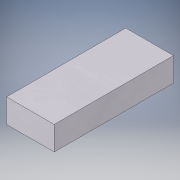
# Autodesk Inventor part: Shaker
Saved by Autodesk Inventor 2017 (Build 210142000, 142)
## iProperties
Created: 2016-12-09
Part Number: Shaker
Material: Aluminum 6061, Welded
Document SubType Name: Modeling
Designer: qupec
Density: 2.7 g/cm^3
Appearance: Weld - Aluminum
Author: qupec
Autodesk Inventor part; units mm, degrees
ref_plane "YZ Plane" through (0, 0, 0) normal (1, 0, 0) x (0, 1, 0)
ref_plane "XZ Plane" through (0, 0, 0) normal (0, 1, 0) x (-1, 0, 0)
ref_plane "XY Plane" through (0, 0, 0) normal (0, 0, 1) x (1, 0, 0)
sketch "Sketch1" plane through (0, 0, 0) normal (0, 1, 0) x (-1, 0, 0)
  line L0 (3, 7.5) -> (-3, 7.5)
  line L1 (-3, 7.5) -> (-3, -7.5)
  line L2 (-3, -7.5) -> (3, -7.5)
  line L3 (3, -7.5) -> (3, 7.5)
  point P0 (0, 0)
  dimension "d0" = 15
  dimension "d1" = 6
  dimension "d2" = 3
  dimension "d3" = 7.5
  constraints: 8 end point, 2 parallel, 1 horizontal, 1 perpendicular
  measures "d0" distance of L2.end L0.start
  measures "d1" distance of L0.start L0.end
  measures "d2" distance from line of point (0, 0) L1
  measures "d3" distance from line of point (0, 0) L0
extrude "Extrusion1" add sketch "Sketch1" along normal blind 3
equation "\"d2\" = 0.5 * d1"
equation "\"d3\" = 0.5 * d0"
body "Solid1"
